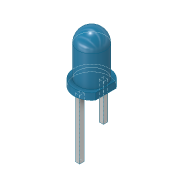
# Autodesk Inventor part: LED
Saved by Autodesk Inventor 2017 (Build 210142000, 142)
## iProperties
Created: 2016-08-05
Part Number: LED
Material: Generic
Document SubType Name: Modeling
Designer: ge937963
Density: 1 g/cm^3
Appearance: Sky Blue Dark
Author: ge937963
Autodesk Inventor part; units mm, degrees
ref_plane "YZ Plane" through (0, 0, 0) normal (1, 0, 0) x (0, 1, 0)
ref_plane "XZ Plane" through (0, 0, 0) normal (0, 1, 0) x (-1, 0, 0)
ref_plane "XY Plane" through (0, 0, 0) normal (0, 0, 1) x (1, 0, 0)
sketch "Sketch1" plane through (0, 0, 0) normal (0, 0, 1) x (1, 0, 0)
  line L0 (0, 0) -> (1.8733, 0)
  line L1 (1.8733, 0) -> (1.8733, 0.7112)
  line L2 (1.8733, 0.7112) -> (1.4478, 0.7112)
  line L3 (1.4478, 0.7112) -> (1.4478, 4.0005)
  arc A0 (1.4478, 4.0005) -> (0, 5.4483) centre (0, 4.0005) ccw
  line L4 (0, 5.4483) -> (0, 0)
  dimension "d0" = 1.4478
  dimension "d1" = 0.7112
  dimension "d2" = 1.8733
  dimension "d3" = 5.4483
  constraints: 10 end point, 3 perpendicular, 2 point on circle, 1 centre point, 1 horizontal, 1 point on line, 1 tangent, 1 vertical
  measures "d0" distance between parallel lines of L4 L3
  measures "d1" distance of L0.end L1.end
  measures "d2" distance between parallel lines of L4 L1
  measures "d3" distance of L0.start L4.start
revolve "Revolution1" add sketch "Sketch1" angle 360 about axis through (0, 5.4483, 0) along (0, -1, 0)
sketch "Sketch2" plane through (0, 0, 0) normal (0, -1, 0) x (1, 0, 0)
  line L0 (4.2518, 2.7248) -> (1.5176, 2.7248)
  line L1 (1.5176, 2.7248) -> (1.5177, -2.7614)
  line L2 (1.5177, -2.7614) -> (4.2518, -2.7614)
  line L3 (4.2518, -2.7614) -> (4.2518, 2.7248)
  circle A0 centre (0, 0) radius 1.8732 projected
  dimension "d5" = 3.3909
  constraints: 8 end point, 2 parallel, 1 horizontal, 1 perpendicular
extrude "Extrusion1" cut sketch "Sketch2" against normal blind 25.4 contours L3 L2 L1 A0 L0 | A0 L1 picked at (1.5825, -0.2532)
sketch "Sketch3" plane through (0, 0, 0) normal (0, -1, 0) x (1, 0, 0)
  line L0 (-0.2286, -1.0287) -> (0.2286, -1.0287)
  line L1 (0.2286, -1.0287) -> (0.2286, -1.5113)
  line L2 (0.2286, -1.5113) -> (-0.2286, -1.5113)
  line L3 (-0.2286, -1.5113) -> (-0.2286, -1.0287)
  line L4 (-0.2286, 1.5113) -> (0.2286, 1.5113)
  line L5 (0.2286, 1.5113) -> (0.2286, 1.0287)
  line L6 (0.2286, 1.0287) -> (-0.2286, 1.0287)
  line L7 (-0.2286, 1.0287) -> (-0.2286, 1.5113)
  line L8 (0, 0) -> (0, 1.0287)
  line L9 (0, 0) -> (0, -1.0287)
  dimension "d13" = 0.4572
  dimension "d14" = 0.4826
  dimension "d15" = 3.0226
  constraints: 20 end point, 4 parallel, 3 equal length, 3 perpendicular, 2 horizontal, 2 midpoint, 1 point on line, 1 vertical alignment
  measures "d13" distance of L1.end L2.end
  measures "d14" distance of L0.end L1.end
  measures "d15" distance between parallel lines of L2 L4
extrude "Extrusion2" add sketch "Sketch3" along normal blind 6.35
sketch "Sketch5" plane through (0.2286, -6.35, -1.0287) normal (1, 0, 0) x (0, 0, -1)
  line L0 (1.6967, -0.6432) -> (-0.5604, -0.6432)
  line L1 (-0.5604, -0.6432) -> (-0.5604, 2.3982)
  line L2 (-0.5604, 2.3982) -> (1.6967, 2.3982)
  line L3 (1.6967, 2.3982) -> (1.6967, -0.6432)
  point P0 (-1.0287, 6.35)
  constraints: 8 end point, 2 parallel, 1 horizontal, 1 perpendicular
extrude "Extrusion3" cut sketch "Sketch5" against normal blind 25.4
body "Solid1"
